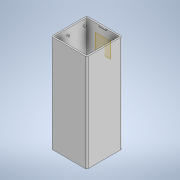
# Autodesk Inventor part: 180caseMain
Saved by Autodesk Inventor 2022 (Build 260153000, 153)
## iProperties
Created: 2022-03-13
Part Number: 180caseMain
Material: Generic
Document SubType Name: Modeling
Designer: maksym
Density: 1 g/cm^3
Appearance: Default
Author: maksym
Autodesk Inventor part; units mm, degrees
ref_plane "YZ Plane" through (0, 0, 0) normal (1, 0, 0) x (0, 1, 0)
ref_plane "XZ Plane" through (0, 0, 0) normal (0, 1, 0) x (-1, 0, 0)
ref_plane "XY Plane" through (0, 0, 0) normal (0, 0, 1) x (1, 0, 0)
sketch "Sketch1" plane through (0, 0, 0) normal (0, 1, 0) x (-1, 0, 0)
  line L0 (0, 0) -> (50, 0)
  line L1 (50, 0) -> (50, -50)
  line L2 (50, -50) -> (0, -50)
  line L3 (0, -50) -> (0, 0)
  dimension "d0" = 50
  dimension "d1" = 50
  constraints: 8 end point, 2 parallel, 1 horizontal, 1 perpendicular
  measures "d0" distance of L1.end L2.end
  measures "d1" distance of L0.end L1.end
extrude "Extrusion1" add sketch "Sketch1" along normal blind 2
sketch "Sketch2" plane through (0, 2, 0) normal (0, 1, 0) x (1, 0, 0)
  line L0 (-48, 2) -> (-2, 2)
  line L1 (-2, 2) -> (-2, 48)
  line L2 (-2, 48) -> (-48, 48)
  line L3 (-48, 48) -> (-48, 2)
  line L4 (0, 50) -> (-50, 50) projected
  line L5 (-50, 50) -> (-50, 0) projected
  line L6 (-50, 0) -> (0, 0) projected
  line L7 (0, 0) -> (0, 50) projected
  dimension "d4" = 2
  dimension "d5" = 2
  dimension "d6" = 2
  dimension "d7" = 2
  constraints: 8 end point, 2 parallel, 1 horizontal, 1 perpendicular
  measures "d4" distance between parallel lines of L4 L2
  measures "d5" distance between parallel lines of L5 L3
  measures "d6" distance between parallel lines of L6 L0
  measures "d7" distance between parallel lines of L7 L1
extrude "Extrusion2" add sketch "Sketch2" along normal blind 135
fillet "Fillet1" radius 2 4 edges at (0, 68.5, 0) (0, 68.5, -50) (-50, 68.5, -50) (-50, 68.5, 0)
sketch "Sketch3" plane through (-2, 2, -48) normal (-1, 0, 0) x (0, 0, 1)
  circle A0 centre (4, 127) radius 1.25
  line L0 (0, 135) -> (46, 135) projected
  line L1 (0, -2) -> (0, 135) projected
  circle A1 centre (4, 94.5) radius 1.25
  circle A2 centre (24, 127) radius 1.25
  circle A3 centre (24, 94.5) radius 1.25
  point P0 (48, -2)
  dimension "d11" = 2.5
  dimension "d14" = 8
  dimension "d15" = 4
  dimension "d16" = 2.5
  dimension "d17" = 32.5
  dimension "d18" = 2.5
  dimension "d19" = 20
  dimension "d20" = 2.5
  dimension "d23" = 32.5
  dimension "d24" = 8
  dimension "d25" = 20
  constraints: 4 centre point
  measures "d11" diameter of A0
  measures "d14" distance from line of L0 A0.centre
  measures "d15" distance from line of A0.centre L1
  measures "d16" diameter of A1
  measures "d17" distance of A0.centre A1.centre
  measures "d18" diameter of A2
  measures "d19" distance of A2.centre A0.centre
  measures "d20" diameter of A3
  measures "d23" distance of A2.centre A3.centre
  measures "d24" distance from line of L0 A2.centre
  measures "d25" distance of A3.centre A1.centre
extrude "Extrusion3" add sketch "Sketch3" along normal blind 2
sketch "Sketch4" plane through (-48, 2, -2) normal (1, 0, 0) x (0, 0, -1)
  circle A0 centre (42, 127) radius 1.25
  line L0 (0, 135) -> (46, 135) projected
  line L1 (46, 135) -> (46, -2) projected
  circle A1 centre (42, 69) radius 1.25
  circle A2 centre (19, 127) radius 1.25
  circle A3 centre (19, 69) radius 1.25
  point P0 (-2, -2)
  dimension "d26" = 2.5
  dimension "d27" = 8
  dimension "d28" = 4
  dimension "d29" = 2.5
  dimension "d30" = 4
  dimension "d31" = 58
  dimension "d32" = 2.5
  dimension "d33" = 8
  dimension "d34" = 23
  dimension "d35" = 2.5
  dimension "d36" = 58
  dimension "d37" = 23
  constraints: 4 centre point
  measures "d26" diameter of A0
  measures "d27" distance from line of L0 A0.centre
  measures "d28" distance from line of L1 A0.centre
  measures "d29" diameter of A1
  measures "d30" distance from line of A1.centre L1
  measures "d31" distance of A1.centre A0.centre
  measures "d32" diameter of A2
  measures "d33" distance from line of L0 A2.centre
  measures "d34" distance of A0.centre A2.centre
  measures "d35" diameter of A3
  measures "d36" distance of A3.centre A2.centre
  measures "d37" distance of A3.centre A1.centre
extrude "Extrusion4" add sketch "Sketch4" along normal blind 2
sketch "Sketch5" plane through (-48, 2, -48) normal (0, 0, 1) x (1, 0, 0)
  line L0 (46, 135) -> (0, 135) construction
  line L1 (46, 0) -> (46, 135) projected
  line L2 (0, 135) -> (46, 135)
  line L3 (23, 135) -> (23, 133) construction
  line L4 (23, 133) -> (28, 133)
  line L5 (23, 133) -> (18, 133)
  line L6 (18, 133) -> (24.2185, 133)
  line L7 (18, 133) -> (18, 135)
  line L8 (28, 133) -> (28, 135)
  point P0 (48, -2)
  dimension "d40" = 2
  dimension "d41" = 5
  dimension "d51" = 5
  constraints: 14 end point, 4 perpendicular, 3 point on line, 1 horizontal, 1 midpoint, 1 vertical
  measures "d40" distance of L3.start L3.end
  measures "d41" distance of L3.end L4.end
  measures "d51" distance of L5.end L3.end
extrude "Extrusion5" add sketch "Sketch5" along normal blind 1
chamfer "Chamfer1" distance 1 angle 45 1 edges at (-25, 137, -47)
ref_plane "Work Plane1" through (-2, 137, -25) normal (0, 0, 1) x (1, 0, 0)
mirror "Mirror1" about plane through (-2, 137, -25) normal (0, 0, 1) of "Extrusion5"
chamfer "Chamfer2" distance 1 angle 45 1 edges at (-25, 137, -3)
fillet "Fillet2" radius 0.5 4 edges at (-25, 136, -47) (-25, 135, -47) (-25, 135, -3) (-25, 136, -3)
body "Solid1"
